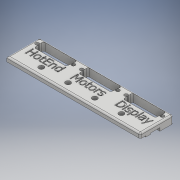
# Autodesk Inventor part: Eletronica - Com25pin
Saved by Autodesk Inventor 2017 (Build 210142000, 142)
## iProperties
Created: 2020-08-30
Part Number: Eletronica - Com25pin
Material: Generic
Document SubType Name: Modeling
Designer: ale
Density: 1 g/cm^3
Appearance: Default
Author: ale
Autodesk Inventor part; units mm, degrees
note: some values were not read from the file. Chosen so that the rebuilt part matches the saved one: direction of "Emboss1".
ref_plane "YZ Plane" through (0, 0, 0) normal (1, 0, 0) x (0, 1, 0)
ref_plane "XZ Plane" through (0, 0, 0) normal (0, 1, 0) x (-1, 0, 0)
ref_plane "XY Plane" through (0, 0, 0) normal (0, 0, 1) x (1, 0, 0)
sketch "Sketch1" plane through (0, 0, 0) normal (0, 0, 1) x (1, 0, 0)
  line L0 (19.5024, 6.36) -> (-19.5024, 6.36)
  arc A0 (-19.5024, 6.36) -> (-21.4937, 4.1742) centre (-19.5024, 4.36) ccw
  line L1 (-21.4937, 4.1742) -> (-20.6803, -4.5458)
  arc A1 (-20.6803, -4.5458) -> (-18.6889, -6.36) centre (-18.6889, -4.36) ccw
  line L2 (-18.6889, -6.36) -> (18.6889, -6.36)
  arc A2 (18.6889, -6.36) -> (20.6803, -4.5458) centre (18.6889, -4.36) ccw
  line L3 (20.6803, -4.5458) -> (21.4937, 4.1742)
  arc A3 (21.4937, 4.1742) -> (19.5024, 6.36) centre (19.5024, 4.36) ccw
  line L4 (-28.5, 8.5) -> (142.5, 8.5)
  line L5 (142.5, -8.5) -> (-28.5, -8.5)
  line L6 (-28.5, -8.5) -> (-28.5, 8.5)
  arc A4 (-21.1884, 0.9013) -> (-21.0573, -0.5045) centre (-23.25, 0) ccw
  arc A5 (21.0573, -0.5045) -> (21.1884, 0.9013) centre (23.25, 0) ccw
  line L7 (76.5024, 6.36) -> (37.4976, 6.36)
  arc A6 (37.4976, 6.36) -> (35.5063, 4.1742) centre (37.4976, 4.36) ccw
  line L8 (35.5063, 4.1742) -> (36.3197, -4.5458)
  arc A7 (36.3197, -4.5458) -> (38.3111, -6.36) centre (38.3111, -4.36) ccw
  line L9 (38.3111, -6.36) -> (75.6889, -6.36)
  arc A8 (75.6889, -6.36) -> (77.6803, -4.5458) centre (75.6889, -4.36) ccw
  line L10 (77.6803, -4.5458) -> (78.4937, 4.1742)
  arc A9 (78.4937, 4.1742) -> (76.5024, 6.36) centre (76.5024, 4.36) ccw
  arc A10 (35.8116, 0.9013) -> (35.9427, -0.5045) centre (33.75, 0) ccw
  arc A11 (78.0573, -0.5045) -> (78.1884, 0.9013) centre (80.25, 0) ccw
  line L11 (133.5024, 6.36) -> (94.4976, 6.36)
  arc A12 (94.4976, 6.36) -> (92.5063, 4.1742) centre (94.4976, 4.36) ccw
  line L12 (92.5063, 4.1742) -> (93.3197, -4.5458)
  arc A13 (93.3197, -4.5458) -> (95.3111, -6.36) centre (95.3111, -4.36) ccw
  line L13 (95.3111, -6.36) -> (132.6889, -6.36)
  arc A14 (132.6889, -6.36) -> (134.6803, -4.5458) centre (132.6889, -4.36) ccw
  line L14 (134.6803, -4.5458) -> (135.4937, 4.1742)
  arc A15 (135.4937, 4.1742) -> (133.5024, 6.36) centre (133.5024, 4.36) ccw
  line L15 (142.5, 8.5) -> (142.5, -8.5)
  arc A16 (92.8116, 0.9013) -> (92.9427, -0.5045) centre (90.75, 0) ccw
  arc A17 (135.0573, -0.5045) -> (135.1884, 0.9013) centre (137.25, 0) ccw
  point P0 (19.6, -5.36)
  point P1 (-19.6, -5.36)
  point P2 (76.6, -5.36)
  point P3 (37.4, -5.36)
  point P4 (133.6, -5.36)
  point P5 (94.4, -5.36)
  dimension "d2" = 39.2
  dimension "d15" = 39.2
  dimension "d18" = 39.2
  dimension "d20" = 17
  constraints: 36 point on circle, 32 end point, 18 centre point, 12 point on line, 4 parallel, 1 horizontal
  measures "d2" distance of point (19.6, -5.36) point (-19.6, -5.36)
  measures "d15" distance of point (76.6, -5.36) point (37.4, -5.36)
  measures "d18" distance of point (133.6, -5.36) point (94.4, -5.36)
  measures "d20" distance of L5.start L4.end
extrude "Extrusion2" add sketch "Sketch1" along normal blind 10
sketch "Sketch3" plane through (0, 0, 10) normal (0, 0, 1) x (1, 0, 0)
  line L0 (-28.5, -8.5) -> (142.5, -8.5)
  line L1 (142.5, -8.5) -> (142.5, -33.5)
  line L2 (142.5, -33.5) -> (-28.5, -33.5)
  line L3 (-28.5, -33.5) -> (-28.5, -8.5)
  line L4 (-28.5, 8.5) -> (-28.5, -8.5)
  line L5 (142.5, -8.5) -> (142.5, 8.5) projected
  point P0 (0, 0)
  dimension "d23" = 171
  dimension "d24" = 25
  dimension "d25" = 0
  dimension "d28" = 0
  constraints: 10 end point, 2 parallel, 1 horizontal, 1 perpendicular
  measures "d23" distance of L1.end L2.end
  measures "d24" distance of L0.end L1.end
  measures "d25" distance between parallel lines of L3 L4
  measures "d28" distance between parallel lines of L1 L5
extrude "Extrusion3" add sketch "Sketch3" against normal blind 6
sketch "Sketch4" plane through (0, 0, 4) normal (0, 0, -1) x (-1, 0, 0)
  line L0 (28.5, 8.5) -> (28.5, -33.5) projected
  line L1 (28.5, -26.5) -> (-142.5, -26.5)
  line L2 (-142.5, -8.5) -> (-142.5, -33.5) projected
  line L3 (28.5, -20.5) -> (-142.5, -20.5)
  line L4 (-142.5, -33.5) -> (28.5, -33.5) projected
  line L5 (-142.5, -20.5) -> (-142.5, -26.5)
  line L6 (28.5, -20.5) -> (28.5, -26.5)
  point P0 (0, 0)
  dimension "d29" = 7
  dimension "d30" = 13
  constraints: 8 end point, 3 point on line, 2 horizontal, 1 collinear, 1 vertical
  measures "d29" distance between parallel lines of L4 L1
  measures "d30" distance between parallel lines of L4 L3
extrude "Extrusion4" add sketch "Sketch4" along normal blind 1.5 contours L0 L1 L2 L3
sketch "Sketch5" plane through (0, 0, 2.5) normal (0, 0, -1) x (-1, 0, 0)
  line L0 (-142.5, -20.5) -> (-142.5, -26.5) projected
  line L1 (-142.5, -23.5) -> (28.5, -23.5)
  line L2 (-142.5, -20.5) -> (28.5, -20.5) projected
  line L3 (-57, -20.5) -> (-57, -26.5)
  point P0 (0, 0)
  point P1 (-108.3, -23.5)
  point P2 (-74.1, -23.5)
  point P3 (-5.7, -23.5)
  point P4 (-39.9, -23.5)
  dimension "d33" = 34.2
  dimension "d34" = 68.4
  constraints: 4 end point, 2 midpoint, 2 point on line, 2 symmetric about line, 1 horizontal, 1 vertical
  measures "d33" distance from line of point (-108.3, -23.5) L0
  measures "d34" distance from line of point (-74.1, -23.5) L0
hole "Hole1" at (108.3, -23.5, 2.5) at (74.1, -23.5, 2.5) at (39.9, -23.5, 2.5) at (5.7, -23.5, 2.5) direction (0, 0, 1) diameter 6.5 end through all counterbore diameter 10 counterbore depth 1.5
sketch "Sketch6" plane through (0, 0, 10) normal (0, 0, 1) x (1, 0, 0)
  line L0 (-21.6234, -7.7534) -> (18.5221, -7.7534) construction
  line L1 (18.5221, -7.7534) -> (18.5221, -15.1622) construction
  line L2 (18.5221, -15.1622) -> (-21.6234, -15.1622) construction
  line L3 (-21.6234, -15.1622) -> (-21.6234, -7.7534) construction
  line L4 (35.2012, -7.6149) -> (75.3467, -7.6149) construction
  line L5 (75.3467, -7.6149) -> (75.3467, -15.0237) construction
  line L6 (75.3467, -15.0237) -> (35.2012, -15.0237) construction
  line L7 (35.2012, -15.0237) -> (35.2012, -7.6149) construction
  line L8 (93.4461, -15.4161) -> (93.4461, -8.0073) construction
  line L9 (93.4461, -8.0073) -> (133.5916, -8.0073) construction
  line L10 (133.5916, -8.0073) -> (133.5916, -15.4161) construction
  line L11 (133.5916, -15.4161) -> (93.4461, -15.4161) construction
  line L12 (-13.3495, -18.1991) -> (-14.6785, -18.1991)
  line L13 (-14.6785, -18.1991) -> (-14.6785, -13.3045)
  line L14 (-14.6785, -13.3045) -> (-19.2814, -13.3045)
  line L15 (-19.2814, -13.3045) -> (-19.2814, -18.1991)
  line L16 (-19.2814, -18.1991) -> (-20.6105, -18.1991)
  line L17 (-20.6105, -18.1991) -> (-20.6105, -8.1991)
  line L18 (-20.6105, -8.1991) -> (-19.2814, -8.1991)
  line L19 (-19.2814, -8.1991) -> (-19.2814, -12.1213)
  line L20 (-19.2814, -12.1213) -> (-14.6785, -12.1213)
  line L21 (-14.6785, -12.1213) -> (-14.6785, -8.1991)
  line L22 (-14.6785, -8.1991) -> (-13.3495, -8.1991)
  line L23 (-13.3495, -8.1991) -> (-13.3495, -18.1991)
  spline S0 degree 2 poles (-5.2539, -14.4471) (-5.2539, -16.3434) (-7.0772, -18.4098) (-8.6007, -18.4098) knots 0 0 0 1 2 2 2
  spline S1 degree 2 poles (-8.6007, -18.4098) (-10.1648, -18.4098) (-11.9557, -16.2785) (-11.9557, -14.4471) knots 0 0 0 1 2 2 2
  spline S2 degree 2 poles (-11.9557, -14.4471) (-11.9557, -12.567) (-10.108, -10.4844) (-8.6007, -10.4844) knots 0 0 0 1 2 2 2
  spline S3 degree 2 poles (-8.6007, -10.4844) (-7.0772, -10.4844) (-5.2539, -12.5589) (-5.2539, -14.4471) knots 0 0 0 1 2 2 2
  spline S4 degree 2 poles (-6.5586, -14.4471) (-6.5586, -12.9884) (-7.6202, -11.5703) (-8.6007, -11.5703) knots 0 0 0 1 2 2 2
  spline S5 degree 2 poles (-8.6007, -11.5703) (-9.5813, -11.5703) (-10.651, -12.9884) (-10.651, -14.4471) knots 0 0 0 1 2 2 2
  spline S6 degree 2 poles (-10.651, -14.4471) (-10.651, -15.8653) (-9.5813, -17.3239) (-8.6007, -17.3239) knots 0 0 0 1 2 2 2
  spline S7 degree 2 poles (-8.6007, -17.3239) (-7.6283, -17.3239) (-6.5586, -15.8896) (-6.5586, -14.4471) knots 0 0 0 1 2 2 2
  spline S8 degree 2 poles (-1.6883, -18.345) (-2.7174, -18.345) (-3.8763, -17.17) (-3.8763, -15.8977) knots 0 0 0 1 2 2 2
  line L24 (-3.8763, -15.8977) -> (-3.8763, -11.7405)
  line L25 (-3.8763, -11.7405) -> (-4.7272, -11.7405)
  line L26 (-4.7272, -11.7405) -> (-4.7272, -10.6951)
  line L27 (-4.7272, -10.6951) -> (-3.8763, -10.6951)
  line L28 (-3.8763, -10.6951) -> (-3.8763, -8.5395)
  line L29 (-3.8763, -8.5395) -> (-2.6121, -8.5395)
  line L30 (-2.6121, -8.5395) -> (-2.6121, -10.6951)
  line L31 (-2.6121, -10.6951) -> (-0.2863, -10.6951)
  line L32 (-0.2863, -10.6951) -> (-0.2863, -11.7405)
  line L33 (-0.2863, -11.7405) -> (-2.6121, -11.7405)
  line L34 (-2.6121, -11.7405) -> (-2.6121, -15.3142)
  spline S9 degree 2 poles (-2.6121, -15.3142) (-2.6121, -15.8815) (-2.5716, -16.5054) (-2.4338, -16.7729) knots 0 0 0 1 2 2 2
  spline S10 degree 2 poles (-2.4338, -16.7729) (-2.3203, -17.0079) (-1.8098, -17.2429) (-1.3722, -17.2429) knots 0 0 0 1 2 2 2
  spline S11 degree 2 poles (-1.3722, -17.2429) (-1.0643, -17.2429) (-0.4889, -17.0565) (-0.3592, -16.9998) knots 0 0 0 1 2 2 2
  line L35 (-0.3592, -16.9998) -> (-0.2863, -16.9998)
  line L36 (-0.2863, -16.9998) -> (-0.2863, -18.1343)
  spline S12 degree 2 poles (-0.2863, -18.1343) (-0.6429, -18.2315) (-1.3722, -18.345) (-1.6883, -18.345) knots 0 0 0 1 2 2 2
  line L37 (0.7429, -18.1991) -> (0.7429, -8.1991)
  line L38 (0.7429, -8.1991) -> (6.9989, -8.1991)
  line L39 (6.9989, -8.1991) -> (6.9989, -9.3823)
  line L40 (6.9989, -9.3823) -> (2.0719, -9.3823)
  line L41 (2.0719, -9.3823) -> (2.0719, -12.1213)
  line L42 (2.0719, -12.1213) -> (6.6667, -12.1213)
  line L43 (6.6667, -12.1213) -> (6.6667, -13.3045)
  line L44 (6.6667, -13.3045) -> (2.0719, -13.3045)
  line L45 (2.0719, -13.3045) -> (2.0719, -17.016)
  line L46 (2.0719, -17.016) -> (6.9989, -17.016)
  line L47 (6.9989, -17.016) -> (6.9989, -18.1991)
  line L48 (6.9989, -18.1991) -> (0.7429, -18.1991)
  line L49 (14.2518, -18.1991) -> (12.9876, -18.1991)
  line L50 (12.9876, -18.1991) -> (12.9876, -13.9204)
  spline S13 degree 2 poles (12.9876, -13.9204) (12.9876, -13.4017) (12.8904, -12.5103) (12.7445, -12.2429) knots 0 0 0 1 2 2 2
  spline S14 degree 2 poles (12.7445, -12.2429) (12.5905, -11.9593) (12.0395, -11.6837) (11.5694, -11.6837) knots 0 0 0 1 2 2 2
  spline S15 degree 2 poles (11.5694, -11.6837) (11.0994, -11.6837) (10.1027, -12.1862) (9.6245, -12.5913) knots 0 0 0 1 2 2 2
  line L51 (9.6245, -12.5913) -> (9.6245, -18.1991)
  line L52 (9.6245, -18.1991) -> (8.3604, -18.1991)
  line L53 (8.3604, -18.1991) -> (8.3604, -10.6951)
  line L54 (8.3604, -10.6951) -> (9.6245, -10.6951)
  line L55 (9.6245, -10.6951) -> (9.6245, -11.5298)
  spline S16 degree 2 poles (9.6245, -11.5298) (10.1918, -11.0192) (11.2858, -10.4844) (11.9017, -10.4844) knots 0 0 0 1 2 2 2
  spline S17 degree 2 poles (11.9017, -10.4844) (13.0038, -10.4844) (14.2518, -11.943) (14.2518, -13.3288) knots 0 0 0 1 2 2 2
  line L56 (14.2518, -13.3288) -> (14.2518, -18.1991)
  line L57 (21.7963, -18.1991) -> (20.5322, -18.1991)
  line L58 (20.5322, -18.1991) -> (20.5322, -17.4374)
  spline S18 degree 2 poles (20.5322, -17.4374) (20.2404, -17.6805) (19.8109, -18.0046) (19.5192, -18.1424) knots 0 0 0 1 2 2 2
  spline S19 degree 2 poles (19.5192, -18.1424) (19.2518, -18.2721) (18.6764, -18.4098) (18.2955, -18.4098) knots 0 0 0 1 2 2 2
  spline S20 degree 2 poles (18.2955, -18.4098) (17.6797, -18.4098) (16.6424, -17.8993) (16.2777, -17.405) knots 0 0 0 1 2 2 2
  spline S21 degree 2 poles (16.2777, -17.405) (15.913, -16.9106) (15.5079, -15.452) (15.5079, -14.5038) knots 0 0 0 1 2 2 2
  spline S22 degree 2 poles (15.5079, -14.5038) (15.5079, -13.5152) (16.0184, -12.0727) (16.4641, -11.5298) knots 0 0 0 1 2 2 2
  spline S23 degree 2 poles (16.4641, -11.5298) (16.8774, -11.0435) (18.0362, -10.4844) (18.6764, -10.4844) knots 0 0 0 1 2 2 2
  spline S24 degree 2 poles (18.6764, -10.4844) (19.2356, -10.4844) (20.0703, -10.7356) (20.5322, -10.9949) knots 0 0 0 1 2 2 2
  line L59 (20.5322, -10.9949) -> (20.5322, -7.7534)
  line L60 (20.5322, -7.7534) -> (21.7963, -7.7534)
  line L61 (21.7963, -7.7534) -> (21.7963, -18.1991)
  line L62 (20.5322, -16.3758) -> (20.5322, -12.0403)
  spline S25 degree 2 poles (20.5322, -12.0403) (20.0621, -11.8134) (19.3166, -11.6432) (18.8871, -11.6432) knots 0 0 0 1 2 2 2
  spline S26 degree 2 poles (18.8871, -11.6432) (17.9147, -11.6432) (16.8126, -13.1019) (16.8126, -14.4795) knots 0 0 0 1 2 2 2
  spline S27 degree 2 poles (16.8126, -14.4795) (16.8126, -15.8085) (17.6553, -17.2105) (18.5873, -17.2105) knots 0 0 0 1 2 2 2
  spline S28 degree 2 poles (18.5873, -17.2105) (19.0816, -17.2105) (20.0865, -16.7567) (20.5322, -16.3758) knots 0 0 0 1 2 2 2
  line L63 (44.7879, -17.6149) -> (43.4589, -17.6149)
  line L64 (43.4589, -17.6149) -> (43.4589, -9.0006)
  line L65 (43.4589, -9.0006) -> (40.8495, -14.8596)
  line L66 (40.8495, -14.8596) -> (40.0391, -14.8596)
  line L67 (40.0391, -14.8596) -> (37.454, -9.0006)
  line L68 (37.454, -9.0006) -> (37.454, -17.6149)
  line L69 (37.454, -17.6149) -> (36.2142, -17.6149)
  line L70 (36.2142, -17.6149) -> (36.2142, -7.6149)
  line L71 (36.2142, -7.6149) -> (38.0294, -7.6149)
  line L72 (38.0294, -7.6149) -> (40.5253, -13.1822)
  line L73 (40.5253, -13.1822) -> (42.9403, -7.6149)
  line L74 (42.9403, -7.6149) -> (44.7879, -7.6149)
  line L75 (44.7879, -7.6149) -> (44.7879, -17.6149)
  spline S29 degree 2 poles (52.8835, -13.8629) (52.8835, -15.7592) (51.0602, -17.8256) (49.5367, -17.8256) knots 0 0 0 1 2 2 2
  spline S30 degree 2 poles (49.5367, -17.8256) (47.9727, -17.8256) (46.1817, -15.6943) (46.1817, -13.8629) knots 0 0 0 1 2 2 2
  spline S31 degree 2 poles (46.1817, -13.8629) (46.1817, -11.9828) (48.0294, -9.9002) (49.5367, -9.9002) knots 0 0 0 1 2 2 2
  spline S32 degree 2 poles (49.5367, -9.9002) (51.0602, -9.9002) (52.8835, -11.9747) (52.8835, -13.8629) knots 0 0 0 1 2 2 2
  spline S33 degree 2 poles (51.5788, -13.8629) (51.5788, -12.4042) (50.5172, -10.9861) (49.5367, -10.9861) knots 0 0 0 1 2 2 2
  spline S34 degree 2 poles (49.5367, -10.9861) (48.5561, -10.9861) (47.4864, -12.4042) (47.4864, -13.8629) knots 0 0 0 1 2 2 2
  spline S35 degree 2 poles (47.4864, -13.8629) (47.4864, -15.281) (48.5561, -16.7397) (49.5367, -16.7397) knots 0 0 0 1 2 2 2
  spline S36 degree 2 poles (49.5367, -16.7397) (50.5091, -16.7397) (51.5788, -15.3053) (51.5788, -13.8629) knots 0 0 0 1 2 2 2
  spline S37 degree 2 poles (56.4492, -17.7608) (55.42, -17.7608) (54.2612, -16.5857) (54.2612, -15.3135) knots 0 0 0 1 2 2 2
  line L76 (54.2612, -15.3135) -> (54.2612, -11.1562)
  line L77 (54.2612, -11.1562) -> (53.4103, -11.1562)
  line L78 (53.4103, -11.1562) -> (53.4103, -10.1109)
  line L79 (53.4103, -10.1109) -> (54.2612, -10.1109)
  line L80 (54.2612, -10.1109) -> (54.2612, -7.9553)
  line L81 (54.2612, -7.9553) -> (55.5253, -7.9553)
  line L82 (55.5253, -7.9553) -> (55.5253, -10.1109)
  line L83 (55.5253, -10.1109) -> (57.8511, -10.1109)
  line L84 (57.8511, -10.1109) -> (57.8511, -11.1562)
  line L85 (57.8511, -11.1562) -> (55.5253, -11.1562)
  line L86 (55.5253, -11.1562) -> (55.5253, -14.73)
  spline S38 degree 2 poles (55.5253, -14.73) (55.5253, -15.2972) (55.5659, -15.9212) (55.7036, -16.1887) knots 0 0 0 1 2 2 2
  spline S39 degree 2 poles (55.7036, -16.1887) (55.8171, -16.4237) (56.3276, -16.6587) (56.7652, -16.6587) knots 0 0 0 1 2 2 2
  spline S40 degree 2 poles (56.7652, -16.6587) (57.0732, -16.6587) (57.6485, -16.4723) (57.7782, -16.4156) knots 0 0 0 1 2 2 2
  line L87 (57.7782, -16.4156) -> (57.8511, -16.4156)
  line L88 (57.8511, -16.4156) -> (57.8511, -17.5501)
  spline S41 degree 2 poles (57.8511, -17.5501) (57.4946, -17.6473) (56.7652, -17.7608) (56.4492, -17.7608) knots 0 0 0 1 2 2 2
  spline S42 degree 2 poles (64.95, -13.8629) (64.95, -15.7592) (63.1266, -17.8256) (61.6031, -17.8256) knots 0 0 0 1 2 2 2
  spline S43 degree 2 poles (61.6031, -17.8256) (60.0391, -17.8256) (58.2482, -15.6943) (58.2482, -13.8629) knots 0 0 0 1 2 2 2
  spline S44 degree 2 poles (58.2482, -13.8629) (58.2482, -11.9828) (60.0958, -9.9002) (61.6031, -9.9002) knots 0 0 0 1 2 2 2
  spline S45 degree 2 poles (61.6031, -9.9002) (63.1266, -9.9002) (64.95, -11.9747) (64.95, -13.8629) knots 0 0 0 1 2 2 2
  spline S46 degree 2 poles (63.6453, -13.8629) (63.6453, -12.4042) (62.5837, -10.9861) (61.6031, -10.9861) knots 0 0 0 1 2 2 2
  spline S47 degree 2 poles (61.6031, -10.9861) (60.6226, -10.9861) (59.5529, -12.4042) (59.5529, -13.8629) knots 0 0 0 1 2 2 2
  spline S48 degree 2 poles (59.5529, -13.8629) (59.5529, -15.281) (60.6226, -16.7397) (61.6031, -16.7397) knots 0 0 0 1 2 2 2
  spline S49 degree 2 poles (61.6031, -16.7397) (62.5756, -16.7397) (63.6453, -15.3053) (63.6453, -13.8629) knots 0 0 0 1 2 2 2
  line L89 (70.2255, -11.4642) -> (70.1607, -11.4642)
  spline S50 degree 2 poles (70.1607, -11.4642) (70.0148, -11.4237) (69.6988, -11.4075) (69.48, -11.4075) knots 0 0 0 1 2 2 2
  spline S51 degree 2 poles (69.48, -11.4075) (68.9694, -11.4075) (67.9646, -11.8532) (67.5108, -12.2908) knots 0 0 0 1 2 2 2
  line L90 (67.5108, -12.2908) -> (67.5108, -17.6149)
  line L91 (67.5108, -17.6149) -> (66.2466, -17.6149)
  line L92 (66.2466, -17.6149) -> (66.2466, -10.1109)
  line L93 (66.2466, -10.1109) -> (67.5108, -10.1109)
  line L94 (67.5108, -10.1109) -> (67.5108, -11.2292)
  spline S52 degree 2 poles (67.5108, -11.2292) (68.1996, -10.6133) (69.2287, -10.1109) (69.715, -10.1109) knots 0 0 0 1 2 2 2
  spline S53 degree 2 poles (69.715, -10.1109) (69.9095, -10.1109) (70.104, -10.1271) (70.2255, -10.1514) knots 0 0 0 1 2 2 2
  line L95 (70.2255, -10.1514) -> (70.2255, -11.4642)
  spline S54 degree 2 poles (73.232, -17.7932) (72.4783, -17.7932) (71.1736, -17.388) (70.7441, -17.1611) knots 0 0 0 1 2 2 2
  line L96 (70.7441, -17.1611) -> (70.7441, -15.743)
  line L97 (70.7441, -15.743) -> (70.809, -15.743)
  spline S55 degree 2 poles (70.809, -15.743) (70.971, -15.8726) (71.4087, -16.1806) (71.7733, -16.3507) knots 0 0 0 1 2 2 2
  spline S56 degree 2 poles (71.7733, -16.3507) (72.0894, -16.5047) (72.8673, -16.7316) (73.2806, -16.7316) knots 0 0 0 1 2 2 2
  spline S57 degree 2 poles (73.2806, -16.7316) (73.5805, -16.7316) (74.2693, -16.5938) (74.4313, -16.4804) knots 0 0 0 1 2 2 2
  spline S58 degree 2 poles (74.4313, -16.4804) (74.6663, -16.3264) (74.877, -15.978) (74.877, -15.6214) knots 0 0 0 1 2 2 2
  spline S59 degree 2 poles (74.877, -15.6214) (74.877, -15.1757) (74.3908, -14.7138) (73.7668, -14.5598) knots 0 0 0 1 2 2 2
  spline S60 degree 2 poles (73.7668, -14.5598) (73.5237, -14.5031) (72.7458, -14.341) (72.4135, -14.2519) knots 0 0 0 1 2 2 2
  spline S61 degree 2 poles (72.4135, -14.2519) (71.5545, -14.0006) (70.7766, -12.9634) (70.7766, -12.2259) knots 0 0 0 1 2 2 2
  spline S62 degree 2 poles (70.7766, -12.2259) (70.7766, -11.2049) (72.3082, -9.9326) (73.5723, -9.9326) knots 0 0 0 1 2 2 2
  spline S63 degree 2 poles (73.5723, -9.9326) (74.1963, -9.9326) (75.4605, -10.2405) (75.89, -10.4755) knots 0 0 0 1 2 2 2
  line L98 (75.89, -10.4755) -> (75.89, -11.8288)
  line L99 (75.89, -11.8288) -> (75.8252, -11.8288)
  spline S64 degree 2 poles (75.8252, -11.8288) (75.339, -11.4399) (74.1558, -10.9942) (73.548, -10.9942) knots 0 0 0 1 2 2 2
  spline S65 degree 2 poles (73.548, -10.9942) (72.924, -10.9942) (72.0651, -11.5209) (72.0651, -12.0477) knots 0 0 0 1 2 2 2
  spline S66 degree 2 poles (72.0651, -12.0477) (72.0651, -12.5258) (72.5756, -12.9877) (73.1428, -13.1335) knots 0 0 0 1 2 2 2
  spline S67 degree 2 poles (73.1428, -13.1335) (73.4184, -13.2065) (74.1153, -13.3524) (74.4962, -13.4415) knots 0 0 0 1 2 2 2
  spline S68 degree 2 poles (74.4962, -13.4415) (75.3228, -13.6522) (76.1655, -14.6165) (76.1655, -15.4512) knots 0 0 0 1 2 2 2
  spline S69 degree 2 poles (76.1655, -15.4512) (76.1655, -15.9374) (75.7847, -16.7964) (75.4119, -17.1125) knots 0 0 0 1 2 2 2
  spline S70 degree 2 poles (75.4119, -17.1125) (75.0148, -17.4447) (74.0018, -17.7932) (73.232, -17.7932) knots 0 0 0 1 2 2 2
  spline S71 degree 2 poles (102.344, -13.4611) (102.344, -14.8306) (101.2338, -17.0348) (100.3018, -17.6507) knots 0 0 0 1 2 2 2
  spline S72 degree 2 poles (100.3018, -17.6507) (99.5401, -18.1288) (97.9761, -18.453) (96.7605, -18.453) knots 0 0 0 1 2 2 2
  line L100 (96.7605, -18.453) -> (94.459, -18.453)
  line L101 (94.459, -18.453) -> (94.459, -8.453)
  line L102 (94.459, -8.453) -> (96.7362, -8.453)
  spline S73 degree 2 poles (96.7362, -8.453) (98.1462, -8.453) (99.7508, -8.8744) (100.318, -9.2471) knots 0 0 0 1 2 2 2
  spline S74 degree 2 poles (100.318, -9.2471) (101.2824, -9.8873) (102.344, -12.0024) (102.344, -13.4611) knots 0 0 0 1 2 2 2
  spline S75 degree 2 poles (100.9582, -13.4449) (100.9582, -12.2941) (100.1965, -10.6653) (99.4428, -10.2034) knots 0 0 0 1 2 2 2
  spline S76 degree 2 poles (99.4428, -10.2034) (98.908, -9.8873) (97.7005, -9.6037) (96.801, -9.6037) knots 0 0 0 1 2 2 2
  line L103 (96.801, -9.6037) -> (95.7881, -9.6037)
  line L104 (95.7881, -9.6037) -> (95.7881, -17.3022)
  line L105 (95.7881, -17.3022) -> (96.801, -17.3022)
  spline S77 degree 2 poles (96.801, -17.3022) (97.6843, -17.3022) (99.0214, -17.0186) (99.5644, -16.6377) knots 0 0 0 1 2 2 2
  spline S78 degree 2 poles (99.5644, -16.6377) (100.2613, -16.1677) (100.9582, -14.6118) (100.9582, -13.4449) knots 0 0 0 1 2 2 2
  line L106 (104.9777, -18.453) -> (103.7135, -18.453)
  line L107 (103.7135, -18.453) -> (103.7135, -10.9489)
  line L108 (103.7135, -10.9489) -> (104.9777, -10.9489)
  line L109 (104.9777, -10.9489) -> (104.9777, -18.453)
  line L110 (105.0668, -9.7009) -> (103.6325, -9.7009)
  line L111 (103.6325, -9.7009) -> (103.6325, -8.3881)
  line L112 (103.6325, -8.3881) -> (105.0668, -8.3881)
  line L113 (105.0668, -8.3881) -> (105.0668, -9.7009)
  spline S79 degree 2 poles (108.8594, -18.6312) (108.1057, -18.6312) (106.801, -18.2261) (106.3715, -17.9992) knots 0 0 0 1 2 2 2
  line L114 (106.3715, -17.9992) -> (106.3715, -16.581)
  line L115 (106.3715, -16.581) -> (106.4364, -16.581)
  spline S80 degree 2 poles (106.4364, -16.581) (106.5984, -16.7107) (107.036, -17.0186) (107.4007, -17.1888) knots 0 0 0 1 2 2 2
  spline S81 degree 2 poles (107.4007, -17.1888) (107.7167, -17.3427) (108.4947, -17.5697) (108.908, -17.5697) knots 0 0 0 1 2 2 2
  spline S82 degree 2 poles (108.908, -17.5697) (109.2078, -17.5697) (109.8966, -17.4319) (110.0587, -17.3184) knots 0 0 0 1 2 2 2
  spline S83 degree 2 poles (110.0587, -17.3184) (110.2937, -17.1645) (110.5044, -16.816) (110.5044, -16.4594) knots 0 0 0 1 2 2 2
  spline S84 degree 2 poles (110.5044, -16.4594) (110.5044, -16.0137) (110.0182, -15.5518) (109.3942, -15.3979) knots 0 0 0 1 2 2 2
  spline S85 degree 2 poles (109.3942, -15.3979) (109.1511, -15.3411) (108.3731, -15.1791) (108.0409, -15.0899) knots 0 0 0 1 2 2 2
  spline S86 degree 2 poles (108.0409, -15.0899) (107.1819, -14.8387) (106.4039, -13.8014) (106.4039, -13.064) knots 0 0 0 1 2 2 2
  spline S87 degree 2 poles (106.4039, -13.064) (106.4039, -12.0429) (107.9355, -10.7706) (109.1997, -10.7706) knots 0 0 0 1 2 2 2
  spline S88 degree 2 poles (109.1997, -10.7706) (109.8237, -10.7706) (111.0879, -11.0786) (111.5174, -11.3136) knots 0 0 0 1 2 2 2
  line L116 (111.5174, -11.3136) -> (111.5174, -12.6669)
  line L117 (111.5174, -12.6669) -> (111.4526, -12.6669)
  spline S89 degree 2 poles (111.4526, -12.6669) (110.9663, -12.2779) (109.7832, -11.8322) (109.1754, -11.8322) knots 0 0 0 1 2 2 2
  spline S90 degree 2 poles (109.1754, -11.8322) (108.5514, -11.8322) (107.6924, -12.359) (107.6924, -12.8857) knots 0 0 0 1 2 2 2
  spline S91 degree 2 poles (107.6924, -12.8857) (107.6924, -13.3638) (108.203, -13.8257) (108.7702, -13.9716) knots 0 0 0 1 2 2 2
  spline S92 degree 2 poles (108.7702, -13.9716) (109.0458, -14.0445) (109.7427, -14.1904) (110.1235, -14.2795) knots 0 0 0 1 2 2 2
  spline S93 degree 2 poles (110.1235, -14.2795) (110.9501, -14.4902) (111.7929, -15.4546) (111.7929, -16.2893) knots 0 0 0 1 2 2 2
  spline S94 degree 2 poles (111.7929, -16.2893) (111.7929, -16.7755) (111.412, -17.6345) (111.0393, -17.9505) knots 0 0 0 1 2 2 2
  spline S95 degree 2 poles (111.0393, -17.9505) (110.6422, -18.2828) (109.6292, -18.6312) (108.8594, -18.6312) knots 0 0 0 1 2 2 2
  spline S96 degree 2 poles (119.2564, -14.4983) (119.2564, -16.3784) (117.4655, -18.5988) (116.096, -18.5988) knots 0 0 0 1 2 2 2
  spline S97 degree 2 poles (116.096, -18.5988) (115.5368, -18.5988) (114.6778, -18.3395) (114.2321, -18.0721) knots 0 0 0 1 2 2 2
  line L118 (114.2321, -18.0721) -> (114.2321, -21.2163)
  line L119 (114.2321, -21.2163) -> (112.968, -21.2163)
  line L120 (112.968, -21.2163) -> (112.968, -10.9489)
  line L121 (112.968, -10.9489) -> (114.2321, -10.9489)
  line L122 (114.2321, -10.9489) -> (114.2321, -11.735)
  spline S98 degree 2 poles (114.2321, -11.735) (114.7022, -11.3055) (115.8529, -10.7382) (116.5255, -10.7382) knots 0 0 0 1 2 2 2
  spline S99 degree 2 poles (116.5255, -10.7382) (117.814, -10.7382) (119.2564, -12.7803) (119.2564, -14.4983) knots 0 0 0 1 2 2 2
  spline S100 degree 2 poles (117.9517, -14.6442) (117.9517, -13.3557) (117.1333, -11.9376) (116.2176, -11.9376) knots 0 0 0 1 2 2 2
  spline S101 degree 2 poles (116.2176, -11.9376) (115.6827, -11.9376) (114.6778, -12.4157) (114.2321, -12.7885) knots 0 0 0 1 2 2 2
  line L123 (114.2321, -12.7885) -> (114.2321, -17.051)
  spline S102 degree 2 poles (114.2321, -17.051) (114.7265, -17.286) (115.4315, -17.4643) (115.8853, -17.4643) knots 0 0 0 1 2 2 2
  spline S103 degree 2 poles (115.8853, -17.4643) (116.8658, -17.4643) (117.9517, -16.0218) (117.9517, -14.6442) knots 0 0 0 1 2 2 2
  line L124 (121.8577, -18.453) -> (120.5936, -18.453)
  line L125 (120.5936, -18.453) -> (120.5936, -8.0073)
  line L126 (120.5936, -8.0073) -> (121.8577, -8.0073)
  line L127 (121.8577, -8.0073) -> (121.8577, -18.453)
  spline S104 degree 2 poles (127.895, -17.6588) (127.7411, -17.7722) (127.2224, -18.1774) (126.9793, -18.299) knots 0 0 0 1 2 2 2
  spline S105 degree 2 poles (126.9793, -18.299) (126.647, -18.4773) (126.0231, -18.6637) (125.4558, -18.6637) knots 0 0 0 1 2 2 2
  spline S106 degree 2 poles (125.4558, -18.6637) (124.9939, -18.6637) (124.1592, -18.3152) (123.8432, -17.9992) knots 0 0 0 1 2 2 2
  spline S107 degree 2 poles (123.8432, -17.9992) (123.5433, -17.6912) (123.1787, -16.7836) (123.1787, -16.2812) knots 0 0 0 1 2 2 2
  spline S108 degree 2 poles (123.1787, -16.2812) (123.1787, -15.5032) (123.8351, -14.4011) (124.5482, -14.0851) knots 0 0 0 1 2 2 2
  spline S109 degree 2 poles (124.5482, -14.0851) (125.1803, -13.7933) (126.8983, -13.5745) (127.895, -13.5178) knots 0 0 0 1 2 2 2
  line L128 (127.895, -13.5178) -> (127.895, -13.2747)
  spline S110 degree 2 poles (127.895, -13.2747) (127.895, -12.8371) (127.6276, -12.2941) (127.3845, -12.1402) knots 0 0 0 1 2 2 2
  spline S111 degree 2 poles (127.3845, -12.1402) (127.1414, -11.9862) (126.4445, -11.8889) (126.0717, -11.8889) knots 0 0 0 1 2 2 2
  spline S112 degree 2 poles (126.0717, -11.8889) (125.6341, -11.8889) (124.4509, -12.1483) (123.8594, -12.3995) knots 0 0 0 1 2 2 2
  line L129 (123.8594, -12.3995) -> (123.7864, -12.3995)
  line L130 (123.7864, -12.3995) -> (123.7864, -11.111)
  spline S113 degree 2 poles (123.7864, -11.111) (124.1349, -11.0137) (125.4396, -10.7706) (126.0798, -10.7706) knots 0 0 0 1 2 2 2
  spline S114 degree 2 poles (126.0798, -10.7706) (126.8577, -10.7706) (127.9193, -11.0137) (128.3407, -11.3298) knots 0 0 0 1 2 2 2
  spline S115 degree 2 poles (128.3407, -11.3298) (128.754, -11.6377) (129.1592, -12.6183) (129.1592, -13.3233) knots 0 0 0 1 2 2 2
  line L131 (129.1592, -13.3233) -> (129.1592, -18.453)
  line L132 (129.1592, -18.453) -> (127.895, -18.453)
  line L133 (127.895, -18.453) -> (127.895, -17.6588)
  line L134 (127.895, -16.6053) -> (127.895, -14.5227)
  spline S116 degree 2 poles (127.895, -14.5227) (127.4412, -14.5632) (126.0717, -14.7009) (125.6422, -14.8306) knots 0 0 0 1 2 2 2
  spline S117 degree 2 poles (125.6422, -14.8306) (125.1398, -14.9846) (124.4834, -15.6248) (124.4834, -16.192) knots 0 0 0 1 2 2 2
  spline S118 degree 2 poles (124.4834, -16.192) (124.4834, -16.8403) (125.2127, -17.4967) (125.9096, -17.4967) knots 0 0 0 1 2 2 2
  spline S119 degree 2 poles (125.9096, -17.4967) (126.5012, -17.4967) (127.4736, -16.9862) (127.895, -16.6053) knots 0 0 0 1 2 2 2
  line L135 (136.8253, -10.9489) -> (132.7897, -21.2163)
  line L136 (132.7897, -21.2163) -> (131.4364, -21.2163)
  line L137 (131.4364, -21.2163) -> (132.7816, -18.0883)
  line L138 (132.7816, -18.0883) -> (130.0587, -10.9489)
  line L139 (130.0587, -10.9489) -> (131.4201, -10.9489)
  line L140 (131.4201, -10.9489) -> (133.4704, -16.5081)
  line L141 (133.4704, -16.5081) -> (135.5125, -10.9489)
  line L142 (135.5125, -10.9489) -> (136.8253, -10.9489)
  point P0 (0, 0)
  constraints: 6 other
emboss "Emboss1" sketch "Sketch6" operation cut depth 1 direction (0, 0, -1)
fillet "Fillet1" radius 2 7 edges at (142.5, 8.5, 5) (142.5, -33.5, 7) (-28.5, 8.5, 5) (57, 8.5, 10) (57, -33.5, 10) (-28.5, -12.5, 10) (142.5, -12.5, 10)
body "Solid2"
